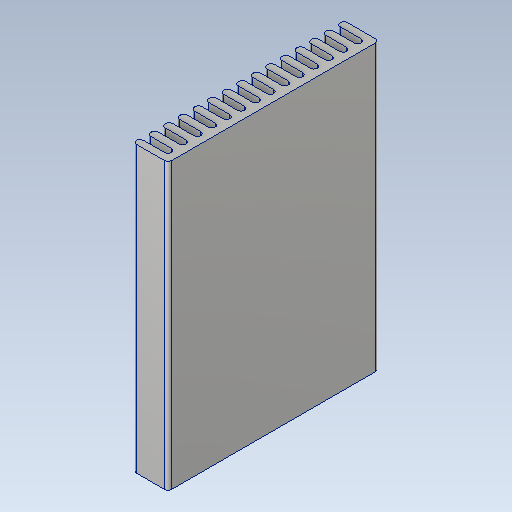
# Autodesk Inventor part: Radiator
Saved by Autodesk Inventor 2020 (Build 240168000, 168)
## iProperties
Created: 2019-01-30
Part Number: Radiator
Material: Aluminium 6061
Document SubType Name: Modeling
Designer: atmat
Density: 2.7 g/cm^3
Appearance: Aluminium — płaski
Mass: 82.0435 g
Surface Area: 281.484 cm^2
Volume: 30.3865 cm^3
Author: atmat
Autodesk Inventor part; units mm, degrees
ref_plane "YZ Plane" through (0, 0, 0) normal (1, 0, 0) x (0, 1, 0)
ref_plane "XZ Plane" through (0, 0, 0) normal (0, 1, 0) x (-1, 0, 0)
ref_plane "XY Plane" through (0, 0, 0) normal (0, 0, 1) x (1, 0, 0)
sketch "Szkic1" plane through (0, 0, 0) normal (0, 1, 0) x (-1, 0, 0)
  line L0 (5, 30) -> (-5, 30)
  line L1 (-5, 30) -> (-5, -30)
  line L2 (-5, -30) -> (5, -30)
  line L3 (5, -30) -> (5, 30)
  point P0 (0, 0)
  dimension "d0" = 10
  dimension "d1" = 5
  dimension "d2" = 60
  dimension "d3" = 30
  constraints: 8 end point, 2 parallel, 1 horizontal, 1 perpendicular
  measures "d0" distance of L1.end L2.end
  measures "d1" distance from line of point (0, 0) L3
  measures "d2" distance of L0.end L1.end
  measures "d3" distance from line of point (0, 0) L2
extrude "Wyciągnięcie proste1" add sketch "Szkic1" along normal blind 100
sketch "Szkic2" plane through (0, 100, 0) normal (0, 1, 0) x (1, 0, 0)
  line L0 (-5, 30) -> (-5, -30) projected
  line L1 (-5, -28) -> (3, -28)
  line L2 (3, -28) -> (3, -26)
  line L3 (3, -26) -> (-5, -26)
  line L4 (-5, -26) -> (-5, -28)
  line L5 (-5, -30) -> (5, -30) projected
  line L6 (5, -30) -> (5, 30) projected
  point P0 (0, 0)
  dimension "d6" = 2
  dimension "d7" = 2
  dimension "d8" = 2
  constraints: 8 end point, 2 parallel, 1 horizontal, 1 perpendicular, 1 point on line
  measures "d6" distance between parallel lines of L3 L1
  measures "d7" distance between parallel lines of L5 L1
  measures "d8" distance between parallel lines of L6 L2
extrude "Wyciągnięcie proste2" cut sketch "Szkic2" against normal blind 100
pattern_linear "Szyk prostokątny1" count 14 spacing 4.15 along (0, 0, -1) of "Wyciągnięcie proste2"
fillet "Zaokrąglenie1" radius 1 2 edges at (-5, 50, 30) (-5, 50, 28)
fillet "Zaokrąglenie2" radius 1 10 edges at (-5, 50, 26) (-5, 50, 23.85) (-5, 50, 21.85) (-5, 50, 19.7) (-5, 50, 17.7) (-5, 50, 15.55) (-5, 50, 13.55) (-5, 50, 11.4) (-5, 50, 9.4) (-5, 50, 7.25)
fillet "Zaokrąglenie3" radius 1 6 edges at (-5, 50, 5.25) (-5, 50, 3.1) (-5, 50, 1.1) (-5, 50, -1.05) (-5, 50, -3.05) (-5, 50, -5.2)
fillet "Zaokrąglenie4" radius 1 12 edges at (-5, 50, -7.2) (-5, 50, -9.35) (-5, 50, -11.35) (-5, 50, -13.5) (-5, 50, -15.5) (-5, 50, -17.65) (-5, 50, -19.65) (-5, 50, -21.8) (-5, 50, -23.8) (-5, 50, -25.95) (-5, 50, -27.95) (-5, 50, -30)
fillet "Zaokrąglenie5" radius 1 16 edges at (3, 50, 28) (3, 50, 26) (3, 50, 23.85) (3, 50, 21.85) (3, 50, 19.7) (3, 50, 17.7) (3, 50, 15.55) (3, 50, 13.55) (3, 50, 11.4) (3, 50, 7.25) (3, 50, 9.4) (3, 50, 5.25) (3, 50, 3.1) (3, 50, 1.1) (3, 50, -1.05) (3, 50, -3.05)
fillet "Zaokrąglenie6" radius 1 12 edges at (3, 50, -5.2) (3, 50, -7.2) (3, 50, -9.35) (3, 50, -11.35) (3, 50, -13.5) (3, 50, -15.5) (3, 50, -17.65) (3, 50, -19.65) (3, 50, -21.8) (3, 50, -23.8) (3, 50, -25.95) (3, 50, -27.95)
fillet "Zaokrąglenie7" radius 1 2 edges at (5, 50, -30) (5, 50, 30)
thicken "Pogrubienie1" operation cut thickness 19 both sides no extend neighbours no toward (0, -1, 0) faces at (4.3333, 100, 3.4667)
